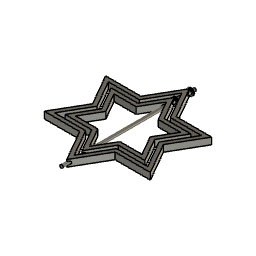
Rotating Star v2 (Autodesk Fusion 360 design; units mm, degrees)
Autodesk Fusion 360 part; units mm, degrees
sketch "Inner Star" plane through (0, 0, 0) normal (0, 0, 1) x (1, 0, 0)
  line L0 (-10, 17.3205) -> (0, 34.641)
  line L1 (0, 34.641) -> (10, 17.3205)
  line L2 (-20, 0) -> (-30, 17.3205)
  line L3 (-30, 17.3205) -> (-10, 17.3205)
  line L4 (-10, -17.3205) -> (-30, -17.3205)
  line L5 (-30, -17.3205) -> (-20, 0)
  line L6 (10, -17.3205) -> (0, -34.641)
  line L7 (0, -34.641) -> (-10, -17.3205)
  line L8 (20, 0) -> (30, -17.3205)
  line L9 (30, -17.3205) -> (10, -17.3205)
  line L10 (10, 17.3205) -> (30, 17.3205)
  line L11 (30, 17.3205) -> (20, 0)
  line L12 (36, 20.7846) -> (24, 0)
  line L13 (0, -41.5692) -> (-12, -20.7846)
  line L14 (12, 20.7846) -> (36, 20.7846)
  line L15 (-24, 0) -> (-36, 20.7846)
  line L16 (0, 41.5692) -> (12, 20.7846)
  line L17 (24, 0) -> (36, -20.7846)
  line L18 (-12, -20.7846) -> (-36, -20.7846)
  line L19 (12, -20.7846) -> (0, -41.5692)
  line L20 (-36, 20.7846) -> (-12, 20.7846)
  line L21 (36, -20.7846) -> (12, -20.7846)
  line L22 (-12, 20.7846) -> (0, 41.5692)
  line L23 (-36, -20.7846) -> (-24, 0)
  dimension "d4" = 360
sketch "Outer Star" plane through (0, 0, 0) normal (0, 0, 1) x (1, 0, 0)
  line L0 (15.96, 27.6435) -> (47.88, 27.6435)
  line L1 (42, -24.2487) -> (14, -24.2487)
  line L2 (-31.92, 0) -> (-47.88, 27.6435)
  line L3 (-14, 24.2487) -> (0, 48.4974)
  line L4 (42, 24.2487) -> (28, 0)
  line L5 (-15.96, 27.6435) -> (0, 55.2871)
  line L6 (-14, -24.2487) -> (-19.6, -24.2487)
  line L7 (-15.96, -27.6435) -> (-47.88, -27.6435)
  line L8 (14, -24.2487) -> (0, -48.4974)
  line L9 (-28, 0) -> (-42, 24.2487)
  line L10 (47.88, -27.6435) -> (15.96, -27.6435)
  line L11 (-47.88, -27.6435) -> (-31.92, 0)
  line L12 (-42, 24.2487) -> (-14, 24.2487)
  line L13 (28, 0) -> (42, -24.2487)
  line L14 (14, 24.2487) -> (42, 24.2487)
  line L15 (-47.88, 27.6435) -> (-15.96, 27.6435)
  line L16 (0, -55.2871) -> (-15.96, -27.6435)
  line L17 (31.92, 0) -> (47.88, -27.6435)
  line L18 (0, 48.4974) -> (14, 24.2487)
  line L19 (0, 55.2871) -> (15.96, 27.6435)
  line L20 (47.88, 27.6435) -> (31.92, 0)
  line L21 (15.96, -27.6435) -> (0, -55.2871)
  line L22 (-42, -24.2487) -> (-28, 0)
  line L23 (0, -48.4974) -> (-14, -24.2487)
  line L24 (-19.6, -24.2487) -> (-42, -24.2487)
sketch "template" plane through (0, 0, 0) normal (0, 0, 1) x (1, 0, 0)
  line L0 (-30, -17.3205) -> (-20, 0)
  line L1 (-10, -17.3205) -> (-30, -17.3205)
  line L2 (36, -20.7846) -> (12, -20.7846)
  line L3 (36, 20.7846) -> (24, 0)
  line L4 (-10, -17.3205) -> (10, -17.3205)
  line L5 (-12, 20.7846) -> (0, 41.5692)
  line L6 (20, 0) -> (30, -17.3205)
  line L7 (10, 17.3205) -> (-10, 17.3205)
  line L8 (0, -34.641) -> (-10, -17.3205)
  line L9 (12, 20.7846) -> (36, 20.7846)
  line L10 (12, -20.7846) -> (24, 0)
  line L11 (12, 20.7846) -> (-12, 20.7846)
  line L12 (-36, -20.7846) -> (-24, 0)
  line L13 (20, 0) -> (10, 17.3205)
  line L14 (10, -17.3205) -> (20, 0)
  line L15 (24, 0) -> (36, -20.7846)
  line L16 (-12, -20.7846) -> (-36, -20.7846)
  line L17 (-24, 0) -> (-12, -20.7846)
  line L18 (30, -17.3205) -> (10, -17.3205)
  line L19 (-20, 0) -> (-10, -17.3205)
  line L20 (-12, -20.7846) -> (12, -20.7846)
  line L21 (12, -20.7846) -> (0, -41.5692)
  line L22 (10, -17.3205) -> (0, -34.641)
  line L23 (0, -41.5692) -> (-12, -20.7846)
  line L24 (30, 17.3205) -> (20, 0)
  line L25 (0, 41.5692) -> (12, 20.7846)
  line L26 (10, 17.3205) -> (30, 17.3205)
  line L27 (-20, 0) -> (-30, 17.3205)
  line L28 (-10, 17.3205) -> (-20, 0)
  line L29 (-12, 20.7846) -> (-24, 0)
  line L30 (-30, 17.3205) -> (-10, 17.3205)
  line L31 (-24, 0) -> (-36, 20.7846)
  line L32 (-36, 20.7846) -> (-12, 20.7846)
  line L33 (0, 34.641) -> (10, 17.3205)
  line L34 (24, 0) -> (12, 20.7846)
  line L35 (-10, 17.3205) -> (0, 34.641)
  dimension "d6" = 360
  constraint parallel L28 L35
  constraint parallel L13 L33
  constraint parallel L5 L29
  constraint parallel L25 L34
sketch "Middle Dowel" plane through (0, 0, 0) normal (0, 1, 0) x (1, 0, 0)
  circle A0 centre (0, -3) radius 1.5
  circle A1 centre (0, -3) radius 1.65
  line L0 (-0.0928, -1.5029) -> (-0.0928, -1.3526)
  line L1 (0.0496, -1.5029) -> (0.0496, -1.3507)
  circle A2 centre (0, -3) radius 3
  dimension "d7" = 3
  dimension "d8" = 3.3
  dimension "d26" = 6
  constraint concentric A0 A1
  constraint coincident A0 L0.start
  constraint coincident A1 L0.end
  constraint vertical L0
  constraint coincident A1 L1.end
  constraint parallel L0 L1
  constraint concentric A1 A2
  measures "d7" diameter of A0
  measures "d8" diameter of A1
  measures "d26" diameter of A2
extrude "Extrude1" add sketch "Outer Star" along normal blind 6 makes body 1
extrude "Extrude2" add sketch "Inner Star" along normal blind 6 separate body makes body 2
extrude "Extrude4" cut sketch "Middle Dowel" along normal blind 60 and the other way blind 60 contours A0 A1 L0 L1 picked at (-0.1721, -1.413) bodies 1 2
extrude "Extrude5" add sketch "Middle Dowel" along normal blind 60 and the other way blind 60 separate body contours A0 makes body 3
extrude "Extrude9" cut sketch "Middle Dowel" along normal blind 5 from surface at 32 contours A0 A1 L0 L1 picked at (0.0338, -1.4505) bodies 2
extrude "Extrude10" cut sketch "Middle Dowel" along normal blind 5 from surface at 48 contours A0 A1 L0 L1 picked at (0.0338, -1.4505) bodies 1
extrude "Extrude11" cut sketch "Middle Dowel" along normal blind 60 and the other way blind 60 contours A0 bodies 1 2
extrude "Extrude12" add sketch "Middle Dowel" along normal blind 1 from surface at 42 separate body contours A0 A1 L0 L1 | A0 A1 L0 L1 | A2 makes body 4
extrude "Extrude13" add sketch "Middle Dowel" along normal blind 1 from surface at 56 separate body contours A0 A1 L0 L1 | A0 A1 L0 L1 | A2 makes body 5
extrude "Extrude14" cut sketch "Middle Dowel" along normal blind 5 from surface at -39 contours A0 A1 L0 L1 picked at (0.0338, -1.4505) bodies 2
extrude "Extrude15" cut sketch "Middle Dowel" along normal blind 5 from surface at -53 contours A0 A1 L0 L1 picked at (0.0338, -1.4505) bodies 1
combine "Combine1" operation add target body 1 tool bodies 2 3 4 5 keep tools result as body 6 in component "Component"
scale "Scale1" factor 1.5 about (20, 0, 0) bodies 6 in component "Component"
extrude "Extrude6" [rolled back] profile offset 43 along distance -1 taper angle 0
extrude "Extrude3" [rolled back] along distance 60 taper angle 0 against distance 60 side2taper angle 0
component "Component" placed x (1, 0, 0) y (0, 1, 0) z (0, 0, 1) at (0, 0, 0)
named bodies: "Outer Star", "Inner Star", "Dowel", "Base 1", "Base 2", "Combined Set Scaled 1.5"
